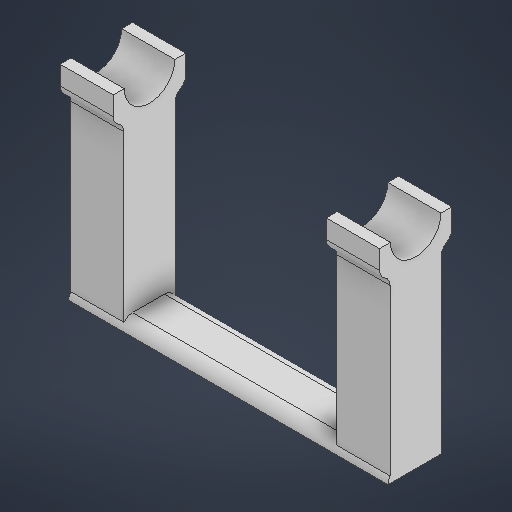
# Autodesk Inventor part: dg_mount
Saved by Autodesk Inventor 2026.1 (Build 301233020, 233B)
## iProperties
Created: 2026-03-05
Part Number: dg_mount
Material: Generic
Document SubType Name: Modeling
Designer: Dylan
Density: 1 g/cm^3
Appearance: Default
Author: Dylan
Autodesk Inventor part; units mm, degrees
ref_plane "YZ Plane" through (0, 0, 0) normal (1, 0, 0) x (0, 1, 0)
ref_plane "XZ Plane" through (0, 0, 0) normal (0, 1, 0) x (-1, 0, 0)
ref_plane "XY Plane" through (0, 0, 0) normal (0, 0, 1) x (1, 0, 0)
sketch "Sketch1" plane through (0, 0, 0) normal (0, 1, 0) x (-1, 0, 0)
  line L0 (0, 0) -> (-60, 0)
  line L1 (-60, 0) -> (-60, 10)
  line L2 (-60, 10) -> (0, 10)
  line L3 (0, 10) -> (0, 0)
  dimension "d0" = 60
  dimension "d1" = 10
  constraints: 8 end point, 2 parallel, 1 horizontal, 1 perpendicular
  measures "d0" distance of L1.end L2.end
  measures "d1" distance of L0.end L1.end
extrude "Extrusion1" add sketch "Sketch1" along normal blind 2
sketch "Sketch2" plane through (0, 2, 0) normal (0, 1, 0) x (1, 0, 0)
  line L0 (0, 0) -> (0, -10) projected
  line L1 (0, 0) -> (10, 0)
  line L2 (10, 0) -> (10, -9.6)
  line L3 (10, -9.6) -> (0, -9.6)
  line L4 (0, -9.6) -> (0, 0)
  line L5 (60, -10) -> (60, 0) projected
  line L6 (60, 0) -> (50, 0)
  line L7 (50, 0) -> (50, -9.6)
  line L8 (50, -9.6) -> (60, -9.6)
  line L9 (60, -9.6) -> (60, 0)
  dimension "d4" = 10
  dimension "d5" = 9.6
  dimension "d6" = 10
  dimension "d7" = 9.6
  constraints: 16 end point, 4 parallel, 2 horizontal, 2 perpendicular
  measures "d4" distance of L2.end L3.end
  measures "d5" distance of L1.end L2.end
  measures "d6" distance of L8.end L7.end
  measures "d7" distance of L7.end L6.end
extrude "Extrusion2" add sketch "Sketch2" along normal blind 37.2
sketch "Sketch3" plane through (0, 2, 9.6) normal (0, 0, 1) x (1, 0, 0)
  line L0 (0, -2) -> (0, 37.2) projected
  line L1 (10, 0) -> (10, 37.2) projected
  line L2 (0, 37.2) -> (10, 37.2)
  line L3 (10, 37.2) -> (10, 32.2)
  line L4 (10, 32.2) -> (0, 32.2)
  line L5 (0, 32.2) -> (0, 37.2)
  line L6 (50, 0) -> (50, 37.2) projected
  line L7 (60, -2) -> (60, 37.2) projected
  line L8 (50, 37.2) -> (60, 37.2)
  line L9 (60, 37.2) -> (60, 32.2)
  line L10 (60, 32.2) -> (50, 32.2)
  line L11 (50, 32.2) -> (50, 37.2)
  point P0 (0, 32.2)
  dimension "d10" = 5
  dimension "d11" = 5
  constraints: 16 end point, 4 parallel, 2 horizontal, 2 perpendicular, 2 point on line
  measures "d10" distance of L2.end L3.end
  measures "d11" distance of L8.end L9.end
extrude "Extrusion3" add sketch "Sketch3" along normal blind 2
sketch "Sketch4" plane through (60, 0, 0) normal (0, 0, -1) x (-1, 0, 0)
  line L0 (0, 0) -> (0, 39.2) projected
  line L1 (10, 2) -> (10, 39.2) projected
  line L2 (0, 39.2) -> (10, 39.2)
  line L3 (10, 39.2) -> (10, 34.2)
  line L4 (10, 34.2) -> (0, 34.2)
  line L5 (0, 34.2) -> (0, 39.2)
  line L6 (50, 2) -> (50, 39.2) projected
  line L7 (60, 0) -> (60, 39.2) projected
  line L8 (50, 39.2) -> (60, 39.2)
  line L9 (60, 39.2) -> (60, 34.2)
  line L10 (60, 34.2) -> (50, 34.2)
  line L11 (50, 34.2) -> (50, 39.2)
  point P0 (0, 34.2)
  dimension "d14" = 5
  dimension "d15" = 5
  constraints: 16 end point, 4 parallel, 2 horizontal, 2 perpendicular, 2 point on line
  measures "d14" distance of L2.end L3.end
  measures "d15" distance of L8.end L9.end
extrude "Extrusion4" add sketch "Sketch4" along normal blind 2
sketch "Sketch5" plane through (0, 0, 0) normal (-1, 0, 0) x (0, 0, 1)
  line L0 (-2, 39.2) -> (11.6, 39.2) projected
  circle A0 centre (4.8, 39.2) radius 4.75
  point P0 (0, 0)
  dimension "d18" = 9.5
  constraints: 1 centre point, 1 midpoint
  measures "d18" diameter of A0
extrude "Extrusion5" cut sketch "Sketch5" against normal through all
fillet "Fillet1" radius 2 8 edges at (55, 34.2, 0) (55, 34.2, 9.6) (55, 34.2, 11.6) (55, 34.2, -2) (5, 34.2, 0) (5, 34.2, -2) (5, 34.2, 9.6) (5, 34.2, 11.6)
fillet "Fillet2" radius 2 2 edges at (30, 2, 10) (30, 2, 0)
body "Solid1"
